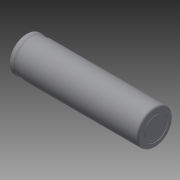
# Autodesk Inventor part: accu_18500
Saved by Autodesk Inventor 2014 (Build 180170000, 170)
## iProperties
Created: 2013-06-25
Part Number: accu_18500
Material: Generisch
Document SubType Name: Modeling
Designer: Felix
Density: 1 g/cm^3
Appearance: Vorgabe
Author: Felix
Autodesk Inventor part; units mm, degrees
ref_plane "YZ Plane" through (0, 0, 0) normal (1, 0, 0) x (0, 1, 0)
ref_plane "XZ Plane" through (0, 0, 0) normal (0, 1, 0) x (-1, 0, 0)
sketch "Skizze1" plane through (0, 0, 0) normal (0, 1, 0) x (-1, 0, 0)
  line L0 (0, 0) -> (67, 0)
  line L1 (67, 0) -> (67, 9.1)
  line L2 (67, 9.1) -> (0, 9.1)
  line L3 (0, 9.1) -> (0, 0)
  line L4 (61, 9.1) -> (64, 9.1)
  line L5 (64, 9.1) -> (64, 8.75)
  line L6 (64, 8.75) -> (61, 8.75)
  line L7 (61, 8.75) -> (61, 9.1)
  line L8 (80.4, 0) -> (-13.4, 0) projected
  dimension "d0" = 67
  dimension "d1" = 9.1
  dimension "d2" = 3
  dimension "d3" = 3
  dimension "d4" = 0.35
  constraints: 16 end point, 4 parallel, 2 horizontal, 2 perpendicular, 1 point on line
  measures "d0" distance of L2.end L1.end
  measures "d1" distance of L1.end L0.end
  measures "d2" distance between parallel lines of L1 L5
  measures "d3" distance of L5.end L6.end
  measures "d4" distance from line of L2 L6.end
revolve "Umdrehung1" add sketch "Skizze1" angle 360 about axis through (-10, 0, 0) along (1, 0, 0) contours L3 L2 L7 L6 L5 L1 L0
ref_plane "Arbeitsebene1" through (-33.5, 0, 0) normal (-1, 0, 0) x (0, 0, 1)
fillet "Rundung1" radius 2 4 edges at (-64, 0, -9.1) (-64, 0, -8.75) (-61, 0, -8.75) (-61, 0, -9.1)
fillet "Rundung2" radius 1 2 edges at (-67, 0, -9.1) (0, 0, -9.1)
sketch "Skizze2" plane through (-67, 0, 0) normal (-1, 0, 0) x (0, 0, 1)
  circle A0 centre (0, 0) radius 8.1 projected
  circle A1 centre (0, 0) radius 6.5
  dimension "d8" = 13
  constraints: 1 centre point, 1 coincident
  measures "d8" diameter of A1
extrude "Extrusion1" cut sketch "Skizze2" against normal blind 0.2 contours A1
mirror "Spiegeln1" about plane through (-33.5, 0, 0) normal (-1, 0, 0) of "Extrusion1"
sketch "Skizze3" plane through (-66.8, 0, 0) normal (-1, 0, 0) x (0, 0, 1)
  circle A0 centre (0, 0) radius 6.5 projected
  circle A1 centre (0, 0) radius 2.85
  dimension "d11" = 5.7
  constraints: 1 centre point, 1 coincident
  measures "d11" diameter of A1
extrude "Extrusion2" add sketch "Skizze3" along normal blind 1 contours A1
fillet "Rundung3" radius 0.5 1 edges at (-67.8, 0, -2.85)
sketch "Skizze4" plane through (-0.2, 0, 0) normal (1, 0, 0) x (0, 0, -1)
  circle A0 centre (0, 0) radius 6.5 projected
  circle A1 centre (0, 0) radius 5.5
  dimension "d15" = 1
  constraints: 1 centre point, 1 coincident
  measures "d15" radial gap between concentric circles of A0 A1
extrude "Extrusion3" add sketch "Skizze4" along normal blind 0.2 contours A1
fillet "Rundung4" radius 0.5 1 edges at (0, 0, 5.5)
